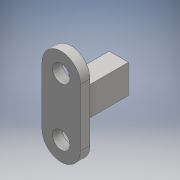
# Autodesk Inventor part: Sztywny uchwyt prowadnic
Saved by Autodesk Inventor 2016 (Build 200138000, 138)
## iProperties
Created: 2018-06-05
Part Number: Sztywny uchwyt prowadnic
Material: Ogólny
Document SubType Name: Modeling
Designer: Agnieszka
Density: 1 g/cm^3
Appearance: Domyślna
Author: Agnieszka
Autodesk Inventor part; units mm, degrees
ref_plane "YZ Plane" through (0, 0, 0) normal (1, 0, 0) x (0, 1, 0)
ref_plane "XZ Plane" through (0, 0, 0) normal (0, 1, 0) x (-1, 0, 0)
ref_plane "XY Plane" through (0, 0, 0) normal (0, 0, 1) x (1, 0, 0)
sketch "Szkic1" plane through (0, 0, 0) normal (0, 1, 0) x (-1, 0, 0)
  circle A0 centre (0, -15) radius 4.5
  circle A1 centre (0, 15) radius 4.5
  line L0 (10, -15) -> (10, 15)
  line L1 (-10, 15) -> (-10, -15)
  arc A2 (10, 15) -> (-10, 15) centre (0, 15) ccw
  arc A3 (-10, -15) -> (10, -15) centre (0, -15) ccw
  point P0 (0, 0)
  dimension "d6" = 9
  constraints: 4 centre point, 4 end point, 4 point on circle, 2 coincident, 2 vertical
  measures "d6" diameter of A0
extrude "Wyciągnięcie proste1" add sketch "Szkic1" along normal blind 5
sketch "Szkic2" plane through (0, 5, 0) normal (0, 1, 0) x (1, 0, 0)
  line L0 (0, -7.5) -> (-10, -7.5)
  line L1 (-10, 15) -> (-10, -15) projected
  line L2 (-10, -7.5) -> (-10, 7.5)
  line L3 (-10, 7.5) -> (10, 7.5)
  line L4 (10, -15) -> (10, 15) projected
  line L5 (0, -7.5) -> (10, -7.5)
  line L6 (10, 7.5) -> (10, -7.5)
  line L7 (0, 0) -> (5, 0)
  line L8 (5, 0) -> (5, 7.5)
  line L9 (5, 0) -> (5, -7.5)
  line L10 (0, 0) -> (-5, 0)
  line L11 (-5, 0) -> (-5, 7.5)
  line L12 (-5, 0) -> (-5, -7.5)
  dimension "d11" = 7.5
  dimension "d12" = 15
  dimension "d13" = 5
  dimension "d14" = 5
  constraints: 22 end point, 8 point on line, 3 perpendicular, 2 midpoint, 1 collinear, 1 horizontal
  measures "d11" distance of L7.start L0.start
  measures "d12" distance of L0.end L2.end
  measures "d13" distance of L7.start L7.end
  measures "d14" distance of L7.start L10.end
extrude "Wyciągnięcie proste2" add sketch "Szkic2" along normal blind 25 contours L0 L12 L10 L7 L9 L5 | L11 L3 L8 L7 L10
